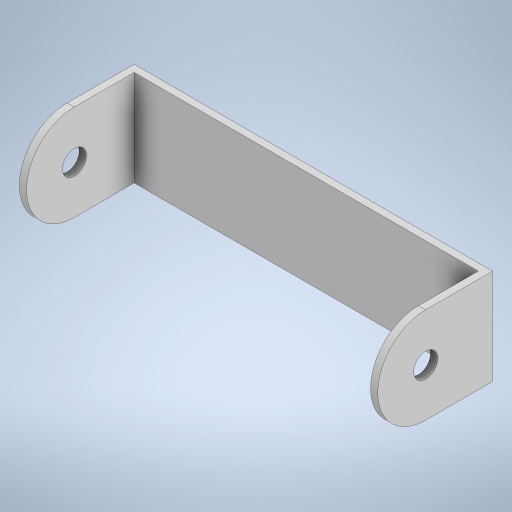
# Autodesk Inventor part: braket
Saved by Autodesk Inventor 2023 (Build 270158000, 158)
## iProperties
Created: 2024-02-06
Part Number: braket
Material: 일반
Document SubType Name: Modeling
Designer: ps737
Density: 1 g/cm^3
Appearance: 기본값
Author: ps737
Autodesk Inventor part; units mm, degrees
ref_plane "YZ Plane" through (0, 0, 0) normal (1, 0, 0) x (0, 1, 0)
ref_plane "XZ Plane" through (0, 0, 0) normal (0, 1, 0) x (-1, 0, 0)
ref_plane "XY Plane" through (0, 0, 0) normal (0, 0, 1) x (1, 0, 0)
sketch "스케치1" plane through (0, 0, 0) normal (0, 0, 1) x (1, 0, 0)
  line L0 (0, 0) -> (150, 0)
  line L1 (150, 0) -> (150, 40)
  line L2 (150, 40) -> (0, 40)
  line L3 (0, 40) -> (0, 0)
  point P0 (150, 20)
  dimension "d0" = 40
  dimension "d1" = 150
  constraints: 8 end point, 2 parallel, 1 horizontal, 1 midpoint, 1 perpendicular
  measures "d0" distance between parallel lines of L0 L2
  measures "d1" distance from line of point (150, 20) L3
extrude "돌출1" add sketch "스케치1" along normal blind 3
sketch "스케치2" plane through (0, 0, 0) normal (-1, 0, 0) x (0, 0, 1)
  line L0 (3, 0) -> (3, 40) projected
  line L1 (3, 40) -> (28.0355, 40)
  line L2 (28.0355, 0) -> (3, 0)
  line L3 (3, 0) -> (3, 40)
  arc A0 (28.0355, 0) -> (28.0355, 40) centre (28.0355, 20) ccw
  circle A1 centre (28.0355, 20) radius 5
  point P0 (0, 0)
  dimension "d5" = 10
  dimension "d6" = 25.0355
  constraints: 6 end point, 2 centre point, 2 point on circle, 2 tangent, 1 coincident, 1 horizontal, 1 perpendicular
  measures "d5" diameter of A1
  measures "d6" distance from line of L1.end L0
extrude "돌출2" add sketch "스케치2" against normal blind 3
sketch "스케치3" plane through (150, 0, 0) normal (1, 0, 0) x (0, 0, -1)
  line L0 (-3, 0) -> (-3, 40) projected
  arc A0 (-28.0355, 40) -> (-28.0355, 0) centre (-28.0355, 20) ccw projected
  line L1 (-3, 0) -> (-28.0355, 0)
  line L2 (0, 40) -> (-28.0355, 40) projected
  line L3 (-28.0355, 40) -> (-3, 40)
  arc A1 (-28.0355, 40) -> (-28.0355, 0) centre (-28.0355, 20) ccw
  circle A2 centre (-28.0355, 20) radius 5 projected
  circle A3 centre (-28.0355, 20) radius 5
  point P0 (0, 0)
  dimension "d10" = 10
  constraints: 4 end point, 2 centre point, 2 coincident, 2 point on circle, 1 horizontal, 1 point on line, 1 tangent
  measures "d10" diameter of A3
extrude "돌출3" add sketch "스케치3" against normal blind 3
